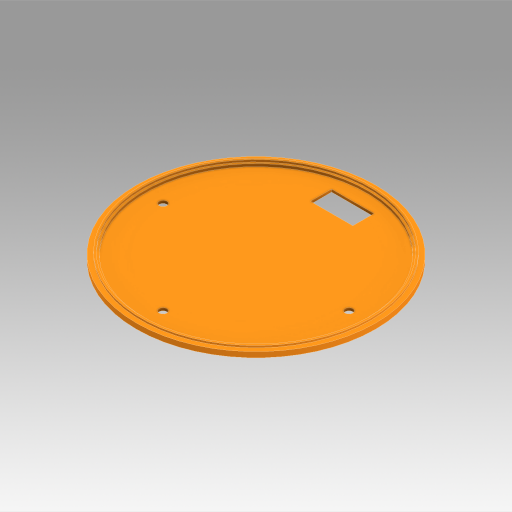
# Autodesk Inventor part: ROUNDTOPCOVER
Saved by Autodesk Inventor 2023 (Build 270158000, 158)
## iProperties
Created: 2025-09-17
Part Number: ROUNDTOPCOVER
Material: Generic
Document SubType Name: Modeling
Designer: NELLY NDUNG'U
Density: 1 g/cm^3
Appearance: Orange
Author: NELLY NDUNG'U
Autodesk Inventor part; units mm, degrees
ref_plane "YZ Plane" through (0, 0, 0) normal (1, 0, 0) x (0, 1, 0)
ref_plane "XZ Plane" through (0, 0, 0) normal (0, 1, 0) x (-1, 0, 0)
ref_plane "XY Plane" through (0, 0, 0) normal (0, 0, 1) x (1, 0, 0)
sketch "Sketch1" plane through (0, 0, 0) normal (0, 1, 0) x (-1, 0, 0)
  circle A0 centre (0, 0) radius 45
  dimension "d0" = 90
  constraints: 1 centre point, 1 coincident
  measures "d0" diameter of A0
extrude "Extrusion1" add sketch "Sketch1" along normal blind 2
sketch "Sketch2" plane through (0, 2, 0) normal (0, 1, 0) x (1, 0, 0)
  circle A0 centre (0, 0) radius 45 projected
  circle A1 centre (0, 0) radius 42.5
  circle A2 centre (0, 0) radius 41.75
  circle A3 centre (0, 0) radius 43.25
  dimension "d3" = 2.5
  dimension "d4" = 0.75
  dimension "d5" = 0.75
  constraints: 3 centre point
  measures "d3" radial gap between concentric circles of A0 A1
  measures "d4" radial gap between concentric circles of A1 A2
  measures "d5" radial gap between concentric circles of A1 A3
extrude "Extrusion2" cut sketch "Sketch2" against normal blind 1 contours A2
extrude "Extrusion3" add sketch "Sketch2" along normal blind 0.75 contours A3
sketch "Sketch3" plane through (0, 1, 0) normal (0, 1, 0) x (1, 0, 0)
  circle A0 centre (0, 0) radius 40 construction
  line L0 (8, 36.45) -> (-8, 36.45)
  line L1 (-8, 36.45) -> (-8, 28.45)
  line L2 (-8, 28.45) -> (8, 28.45)
  line L3 (8, 28.45) -> (8, 36.45)
  circle A1 centre (35, 0) radius 1.5
  circle A2 centre (0, -35) radius 1.5
  circle A3 centre (-35, 0) radius 1.5
  line L4 (40, 0) -> (-40, 0) construction
  line L5 (0, 0) -> (0, -40) construction
  line L6 (0, 0) -> (0, 40) construction
  point P0 (0, 36.45)
  dimension "d10" = 80
  dimension "d11" = 5
  dimension "d12" = 3
  dimension "d13" = 3
  dimension "d14" = 5
  dimension "d15" = 3
  dimension "d16" = 5
  dimension "d17" = 16
  dimension "d18" = 8
  dimension "d21" = 36.45
  constraints: 14 end point, 4 centre point, 4 point on circle, 3 point on line, 2 horizontal, 2 midpoint, 2 parallel, 1 coincident, 1 perpendicular, 1 vertical, 1 other
  measures "d10" diameter of A0
  measures "d11" distance of L4.start A1.centre
  measures "d12" diameter of A1
  measures "d13" diameter of A2
  measures "d14" distance of L5.end A2.centre
  measures "d15" diameter of A3
  measures "d16" distance of L4.end A3.centre
  measures "d17" distance of L1.end L2.end
  measures "d18" distance between parallel lines of L0 L2
  measures "d21" distance from line of L0 point (0, 0)
extrude "Extrusion5" cut sketch "Sketch3" against normal through all contours L3 L2 L1 L0
extrude "Extrusion6" cut sketch "Sketch3" against normal through all contours A1 | A2 | A3
body "Solid1"
